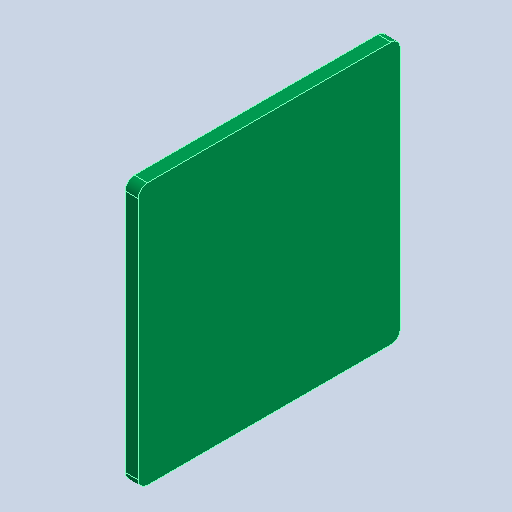
# Autodesk Inventor part: Cover Top (Normal) Proto
Saved by Autodesk Inventor 2023.1 (Build 271208000, 208)
## iProperties
Created: 2023-02-07
Part Number: Cover Top (Normal) Proto
Material: Generic
Document SubType Name: Modeling
Designer: xSibe
Density: 1 g/cm^3
Appearance: Plastic Dark Green
Author: xSibe
Autodesk Inventor part; units mm, degrees
ref_plane "YZ Plane" through (0, 0, 0) normal (1, 0, 0) x (0, 1, 0)
ref_plane "XZ Plane" through (0, 0, 0) normal (0, 1, 0) x (-1, 0, 0)
sketch "Sketch1" plane through (0, 0, 0) normal (1, 0, 0) x (0, 1, 0)
  circle A0 centre (-21.9, 21.9) radius 1.875 projected
  circle A1 centre (21.9, -21.9) radius 1.875 projected
  circle A2 centre (-21.9, -21.9) radius 1.875 projected
  circle A3 centre (21.9, 21.9) radius 1.875 projected
  circle A4 centre (20.8, -14.4) radius 2.0734 projected
  circle A5 centre (-20.8, 14.4) radius 2.0734 projected
  circle A6 centre (-20.8, -14.4) radius 2.0734 projected
  circle A7 centre (-14.4, -20.8) radius 2.0734 projected
  line L0 (17.05, 17.05) -> (-17.05, 17.05) projected
  line L1 (17.05, -17.05) -> (17.05, 17.05) projected
  line L2 (-17.05, -17.05) -> (17.05, -17.05) projected
  line L3 (-17.05, 17.05) -> (-17.05, -17.05) projected
  circle A8 centre (14.4, -20.8) radius 2.0734 projected
  circle A9 centre (20.8, 14.4) radius 2.0734 projected
  circle A10 centre (-14.4, 20.8) radius 2.0734 projected
  circle A11 centre (14.4, 20.8) radius 2.0734 projected
  line L4 (24.875, 22.9) -> (24.875, -22.9) projected
  arc A12 (24.875, 22.9) -> (22.9, 24.875) centre (22.9, 22.9) ccw projected
  line L5 (-22.9, 24.875) -> (22.9, 24.875) projected
  arc A13 (-22.9, 24.875) -> (-24.875, 22.9) centre (-22.9, 22.9) ccw projected
  line L6 (-24.875, -22.9) -> (-24.875, 22.9) projected
  arc A14 (-24.875, -22.9) -> (-22.9, -24.875) centre (-22.9, -22.9) ccw projected
  line L7 (22.9, -24.875) -> (-22.9, -24.875) projected
  arc A15 (22.9, -24.875) -> (24.875, -22.9) centre (22.9, -22.9) ccw projected
  arc A16 (-24.625, -22.9) -> (-22.9, -24.625) centre (-22.9, -22.9) ccw
  line L8 (-24.625, -22.9) -> (-24.625, 22.9)
  arc A17 (-22.9, 24.625) -> (-24.625, 22.9) centre (-22.9, 22.9) ccw
  line L9 (-22.9, 24.625) -> (22.9, 24.625)
  arc A18 (24.625, 22.9) -> (22.9, 24.625) centre (22.9, 22.9) ccw
  line L10 (24.625, 22.9) -> (24.625, -22.9)
  arc A19 (22.9, -24.625) -> (24.625, -22.9) centre (22.9, -22.9) ccw
  line L11 (22.9, -24.625) -> (-22.9, -24.625)
  point P0 (0, 0)
  dimension "d0" = 0.25
  constraints: 8 end point, 8 point on circle, 4 centre point, 7 other
  measures "d0" distance between parallel lines of L7 L11
ref_plane "Work Plane1" through (49.8, -24.875, -24.875) normal (1, 0, 0) x (0, 1, 0)
extrude "Extrusion1" add sketch "Sketch1" along normal blind 2.5 from surface at 49.8 contours A0 | A1 | A2 | A3 | A4 | A5 | A6 | A7 | L1 L2 L3 L0 | A8 | A9 | A10 | A11 | L8 A17 L9 A18 L10 A19 L11 A16
sketch "Sketch2" plane through (52.3, -22.9, -24.625) normal (1, 0, 0) x (0, 0, -1)
  circle A0 centre (-46.525, 1) radius 1.875 projected
  circle A1 centre (-2.725, 44.8) radius 1.875 projected
  circle A2 centre (-2.725, 1) radius 1.875 projected
  circle A3 centre (-46.525, 44.8) radius 1.875 projected
  circle A4 centre (-10.225, 43.7) radius 2.0734 projected
  circle A5 centre (-39.025, 2.1) radius 2.0734 projected
  circle A6 centre (-10.225, 2.1) radius 2.0734 projected
  circle A7 centre (-3.825, 8.5) radius 2.0734 projected
  line L0 (-41.675, 39.95) -> (-41.675, 5.85) projected
  line L1 (-7.575, 39.95) -> (-41.675, 39.95) projected
  line L2 (-7.575, 5.85) -> (-7.575, 39.95) projected
  line L3 (-41.675, 5.85) -> (-7.575, 5.85) projected
  circle A8 centre (-3.825, 37.3) radius 2.0734 projected
  circle A9 centre (-39.025, 43.7) radius 2.0734 projected
  circle A10 centre (-45.425, 8.5) radius 2.0734 projected
  circle A11 centre (-45.425, 37.3) radius 2.0734 projected
  line L4 (-47.525, 47.775) -> (-1.725, 47.775) projected
  arc A12 (-47.525, 47.775) -> (-49.5, 45.8) centre (-47.525, 45.8) ccw projected
  line L5 (-49.5, 0) -> (-49.5, 45.8) projected
  arc A13 (-49.5, 0) -> (-47.525, -1.975) centre (-47.525, 0) ccw projected
  line L6 (-1.725, -1.975) -> (-47.525, -1.975) projected
  arc A14 (-1.725, -1.975) -> (0.25, 0) centre (-1.725, 0) ccw projected
  line L7 (0.25, 45.8) -> (0.25, 0) projected
  arc A15 (0.25, 45.8) -> (-1.725, 47.775) centre (-1.725, 45.8) ccw projected
  line L8 (-41.6, 39.875) -> (-41.6, 5.925)
  line L9 (-41.6, 5.925) -> (-7.65, 5.925)
  line L10 (-7.65, 5.925) -> (-7.65, 39.875)
  line L11 (-7.65, 39.875) -> (-41.6, 39.875)
  line L12 (-40.35, 38.625) -> (-40.35, 7.175)
  line L13 (-40.35, 7.175) -> (-8.9, 7.175)
  line L14 (-8.9, 7.175) -> (-8.9, 38.625)
  line L15 (-8.9, 38.625) -> (-40.35, 38.625)
  dimension "d16" = 0.075
  dimension "d17" = 1.25
  constraints: 16 end point, 6 other
  measures "d16" distance between parallel lines of L1 L11
  measures "d17" distance between parallel lines of L11 L15
extrude "Extrusion2" add sketch "Sketch2" against normal blind 2.5 from surface at -2.5 contours L11 L10 L9 L8
body "Solid1"
